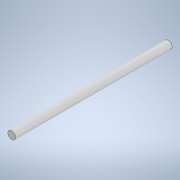
# Autodesk Inventor part: wał2
Saved by Autodesk Inventor 2022 (Build 260153000, 153)
## iProperties
Created: 2023-04-25
Part Number: wał2
Material: Ogólny
Document SubType Name: Modeling
Designer: nosal
Density: 1 g/cm^3
Appearance: Domyślna
Author: nosal
Autodesk Inventor part; units mm, degrees
ref_plane "YZ Plane" through (0, 0, 0) normal (1, 0, 0) x (0, 1, 0)
ref_plane "XZ Plane" through (0, 0, 0) normal (0, 1, 0) x (-1, 0, 0)
ref_plane "XY Plane" through (0, 0, 0) normal (0, 0, 1) x (1, 0, 0)
sketch "Szkic1" plane through (0, 0, 0) normal (0, 0, 1) x (1, 0, 0)
  circle A0 centre (-0.2385, 0) radius 4
  point P0 (0, 0)
  dimension "d0" = 8
  dimension "d0" = 8
  constraints: 1 centre point
  measures "d0" diameter of A0
extrude "Wyciągnięcie proste1" add sketch "Szkic1" along normal blind 160
